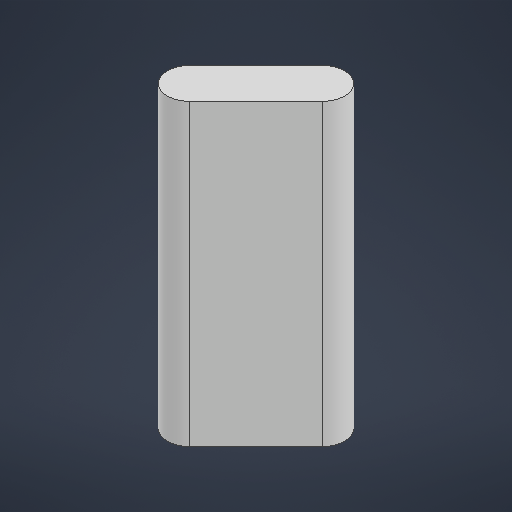
# Autodesk Inventor part: Drone_leg
Saved by Autodesk Inventor 2026.1 (Build 301233000, 233)
## iProperties
Created: 2025-07-29
Part Number: Drone_leg
Material: Generic
Document SubType Name: Modeling
Designer: rohit
Density: 1 g/cm^3
Appearance: Default
Author: rohit
Autodesk Inventor part; units mm, degrees
ref_plane "YZ Plane" through (0, 0, 0) normal (1, 0, 0) x (0, 1, 0)
ref_plane "XZ Plane" through (0, 0, 0) normal (0, 1, 0) x (-1, 0, 0)
ref_plane "XY Plane" through (0, 0, 0) normal (0, 0, 1) x (1, 0, 0)
sketch "Sketch1" plane through (0, 0, 0) normal (0, 1, 0) x (-1, 0, 0)
  circle A0 centre (0.2636, -10.4031) radius 3.175
  line L0 (0.2636, -10.4031) -> (6.9811, -3.6856)
  line L1 (0.2636, -10.4031) -> (6.0619, -16.2014)
  line L2 (0.2636, -10.4031) -> (-5.5347, -4.6048)
  line L3 (0.2636, -10.4031) -> (-6.4539, -17.1206)
  circle A1 centre (6.9811, -3.6856) radius 1.75
  circle A2 centre (6.0619, -16.2014) radius 1.75
  circle A3 centre (-6.4539, -17.1206) radius 1.75
  circle A4 centre (-5.5347, -4.6048) radius 1.75
  circle A5 centre (0.2636, -10.4031) radius 14.1446
  circle A6 centre (6.9811, -3.6856) radius 4.445
  circle A7 centre (-6.4539, -17.1206) radius 4.445
  line L4 (3.838, -0.5425) -> (-9.597, -13.9775)
  line L5 (10.1242, -6.8287) -> (-3.3108, -20.2637)
  circle A8 centre (6.9811, -3.6856) radius 2.3813
  point P0 (0, 0)
  dimension "d3" = 9.5
  dimension "d4" = 90
  dimension "d5" = 90
  dimension "d6" = 90
  dimension "d7" = 3.5
  dimension "d8" = 3.5
  dimension "d9" = 3.5
  dimension "d10" = 3.5
  dimension "d12" = 8.89
  dimension "d13" = 8.89
  dimension "d18" = 4.7625
  constraints: 12 end point, 9 centre point, 7 coincident, 4 point on circle, 2 tangent, 1 point on line
  measures "d3" distance of L0.start L3.end
  measures "d4" angle of L1 L0
  measures "d5" angle of L0 L2
  measures "d6" angle of L2 L3
  measures "d7" diameter of A1
  measures "d8" diameter of A2
  measures "d9" diameter of A3
  measures "d10" diameter of A4
  measures "d12" diameter of A6
  measures "d13" diameter of A7
  measures "d18" diameter of A8
extrude "Extrusion2" add sketch "Sketch1" along normal blind 3.175 contours A0 L0 A6 L5 L1 | A0 L2 L4 A6 L0 | L1 L5 A7 L3 A0 | A0 L3 A7 L4 L2 | A8 | A6 | A7
sketch "Sketch3" plane through (0, 3.175, 0) normal (0, 1, 0) x (1, 0, 0)
  circle A0 centre (-6.9811, 3.6856) radius 1.75 projected
  line L0 (-6.9811, 3.6856) -> (-6.9811, 13.6529)
  arc A1 (-11.4261, 3.6856) -> (-3.838, 0.5425) centre (-6.9811, 3.6856) ccw
  arc A2 (-10.126, 3.2493) -> (-4.7361, 1.4405) centre (-6.9811, 3.6856) ccw
  circle A3 centre (6.4539, 17.1206) radius 1.75 projected
  arc A4 (8.699, 14.8755) -> (6.8902, 20.2655) centre (6.4539, 17.1206) ccw
  arc A5 (9.597, 13.9775) -> (6.4539, 21.5656) centre (6.4539, 17.1206) ccw
  line L1 (-3.838, 0.5425) -> (9.597, 13.9775) projected
  line L2 (-3.838, 0.5425) -> (9.597, 13.9775)
  line L3 (-4.7361, 1.4405) -> (8.699, 14.8755)
  arc A6 (-10.1242, 6.8287) -> (-3.838, 0.5425) centre (-6.9811, 3.6856) ccw projected
  line L4 (6.8902, 20.2655) -> (6.4539, 21.5656)
  line L5 (-10.126, 3.2493) -> (-11.4261, 3.6856)
  point P0 (0, 0)
  constraints: 10 end point, 9 point on circle, 4 centre point, 4 coincident, 2 point on line, 1 tangent, 1 vertical
extrude "Extrusion3" add sketch "Sketch3" along normal blind 25.4 contours L5 A2 L3 A4 L4 A5 L1 A1
sketch "Sketch4" plane through (0, 28.575, 0) normal (0, 1, 0) x (1, 0, 0)
  circle A0 centre (-6.9811, 3.6856) radius 1.75 projected
  circle A1 centre (-6.9811, 3.6856) radius 4.445
  circle A2 centre (6.4539, 17.1206) radius 1.75 projected
  circle A3 centre (6.4539, 17.1206) radius 4.445
  arc A4 (-11.4261, 3.6856) -> (-3.838, 0.5425) centre (-6.9811, 3.6856) ccw projected
  line L0 (-3.838, 0.5425) -> (9.597, 13.9775)
  line L1 (3.3108, 20.2637) -> (-10.1242, 6.8287) projected
  line L2 (-10.1242, 6.8287) -> (3.3108, 20.2637)
  point P0 (0, 0)
  constraints: 4 end point, 3 point on circle, 2 centre point, 2 coincident, 1 collinear, 1 tangent
extrude "Extrusion4" add sketch "Sketch4" along normal blind 31.75 contours A0 | A1 | A1 L1 A3 L0 | A3 | A2
body "Solid2"
